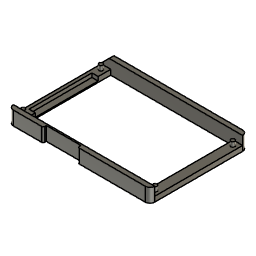
ScreenBezel v5 (Autodesk Fusion 360 design; units mm, degrees)
Autodesk Fusion 360 part; units mm, degrees
sketch "Sketch1" plane through (0, 0, 0) normal (0, 0, 1) x (1, 0, 0)
  line L0 (-50, 25) -> (28, 25)
  line L1 (28, 25) -> (28, -31)
  line L2 (28, -31) -> (-50, -31)
  line L3 (-50, -31) -> (-50, 25)
  line L4 (-55, 30) -> (30, 30)
  line L5 (30, 30) -> (30, -35)
  line L6 (30, -35) -> (-55, -35)
  line L7 (-55, -35) -> (-55, 30)
  dimension "d1" = 78
  dimension "d2" = 56
  constraint horizontal L0
  constraint vertical L1
  constraint horizontal L2
  constraint vertical L3
  constraint horizontal L4
  constraint vertical L5
  constraint horizontal L6
  constraint vertical L7
  measures "d1" distance of L0.start L0.end
  measures "d2" distance of L0.start L2.end
extrude "Extrude1" add sketch "Sketch1" along normal blind 3
sketch "Sketch2" plane through (0, 0, 3) normal (0, 0, 1) x (-1, 0, 0)
  line L0 (-28, 31) -> (50, 31)
  line L1 (50, 31) -> (50, -25)
  line L2 (50, -25) -> (-28, -25)
  line L3 (-28, -25) -> (-28, 31)
  line L4 (55, 35) -> (-30, 35)
  line L5 (-30, 35) -> (-30, -30)
  line L6 (-30, -30) -> (55, -30)
  line L7 (55, -30) -> (55, 35)
  line L8 (50, -25) -> (-28, -25)
  line L9 (-28, -25) -> (-28, -30)
  line L10 (-28, -30) -> (50, -30)
  line L11 (50, -30) -> (50, -25)
  line L12 (-28, 31) -> (50, 31)
  line L13 (50, 31) -> (50, 35)
  line L14 (50, 35) -> (-28, 35)
  line L15 (-28, 35) -> (-28, 31)
  constraint horizontal L8
  constraint vertical L9
  constraint horizontal L10
  constraint vertical L11
  constraint coincident L6 L9.end
  constraint coincident L1.end L2.start
  constraint horizontal L12
  constraint vertical L13
  constraint horizontal L14
  constraint vertical L15
  constraint coincident L4 L13.end
  constraint coincident L0.start L3.end
extrude "Extrude2" add sketch "Sketch2" along normal blind 5 contours L0 L4 L12 L13 L14 L15 | L2 L6 L8 L9 L10 L11
extrude "Extrude3" add 1 faces at (30, 8.3333, 1) along direction (1, 0, 0) blind 4
extrude "Extrude4" add 1 faces at (-55, -13.3333, 1) along direction (-1, 0, 0) blind 1
sketch "Sketch3" plane through (0, 0, 3) normal (0, 0, 1) x (-1, 0, 0)
  line L0 (50, 35) -> (50, 31)
  line L1 (50, 31) -> (50, -25)
  line L2 (50, -25) -> (50, -30)
  line L3 (50, -30) -> (56, -30)
  line L4 (56, -30) -> (56, 35)
  line L5 (56, 35) -> (50, 35)
  circle A0 centre (53, -21.75) radius 1.25
  circle A1 centre (-31, -21.75) radius 1.25
  circle A2 centre (-31, 27.75) radius 1.25
  circle A3 centre (53, 27.75) radius 1.25
  dimension "d11" = 2.5
  dimension "d12" = 2.5
  dimension "d13" = 2.5
  dimension "d14" = 2.5
  measures "d11" diameter of A0
  measures "d12" diameter of A1
  measures "d13" diameter of A2
  measures "d14" diameter of A3
extrude "Extrude5" add sketch "Sketch3" along normal blind 3 contours A0 | A1 | A2 | A3
extrude "Extrude6" add 2 faces at (2, 28.3333, 8) (2, -32.3333, 8) along direction (0, 0, 1) blind 1
extrude "Extrude7" cut 1 faces at (-24, 30, 7) along direction (0, -1, 0) blind 2
extrude "Extrude8" cut 1 faces at (-24, -35, 5) along direction (0, 1, 0) blind 1
sketch "Sketch4" plane through (0, 0, 3) normal (0, 0, 1) x (-1, 0, 0)
  line L0 (56, 34) -> (50, 34)
  line L1 (50, 34) -> (50, 31)
  line L2 (50, 31) -> (50, -25)
  line L3 (50, -25) -> (50, -28)
  line L4 (50, -28) -> (56, -28)
  line L5 (56, -28) -> (56, 34)
  circle A0 centre (53, -21.75) radius 1.25
  circle A1 centre (53, 27.75) radius 1.25
  line L6 (50, -17) -> (54, -17)
  line L7 (54, -17) -> (54, 23)
  line L8 (54, 23) -> (50, 23)
  line L9 (50, 23) -> (50, -17)
  constraint horizontal L6
  constraint vertical L7
  constraint horizontal L8
  constraint vertical L9
  constraint coincident L2 L6.start
extrude "Extrude9" cut sketch "Sketch4" against normal blind 2.5 contours L2 L6 L7 L8 L9
extrude "Extrude10" add 2 faces at (-50, -32, 5) (-50, 26, 5) along direction (-1, 0, 0) up to surface end surface through (-56, -35, 0) normal (-1, 0, 0) offset 0
extrude "Extrude11" add 2 faces at (28, -32, 7) (28, 26, 5) along direction (1, 0, 0) up to surface end surface through (34, 30, 0) normal (1, 0, 0) offset 0
extrude "Extrude12" cut 2 faces at (4, 26, 9) (4, -33, 9) along direction (0, 0, -1) blind 0.5
chamfer "Chamfer1" distance 5 angle 45 1 edges at (-56, 26.5, 8.5)
fillet "Fillet4" radius 3 3 edges at (-56, -34, 4.25) (34, -34, 4.25) (34, 28, 4.25)
sketch "Sketch5" plane through (0, -34, 0) normal (0, -1, 0) x (1, 0, 0)
  line L0 (31, 0) -> (31, 8.5)
  line L1 (31, 8.5) -> (-53, 8.5)
  line L2 (-53, 8.5) -> (-53, 0)
  line L3 (-53, 0) -> (31, 0)
  line L4 (-56, 0) -> (-34, 0)
  line L5 (-34, 0) -> (-34, 10.214)
  line L6 (-34, 10.214) -> (-12, 10.214)
  line L7 (-12, 10.214) -> (-12, -0.4704)
  line L8 (-12, -0.4704) -> (-34, -0.4704)
  line L9 (-34, -0.4704) -> (-34, 0)
  point P0 (-56, 0)
  dimension "d40" = 90
  dimension "d41" = 22
  constraint coincident P0 L4.start
  constraint coincident L3 L4.end
  constraint perpendicular L5 L6
  constraint perpendicular L3 L7
  constraint perpendicular L5 L8
  constraint perpendicular L3 L9
  measures "d40" angle of L4 L5
  measures "d41" distance of L5.end L6.end
extrude "Extrude13" cut sketch "Sketch5" against normal blind 2 contours L1 L3 L5 L7
fillet "Fillet5" radius 1 2 edges at (-34, -34, 4.25) (-12, -34, 4.25)
extrude "Extrude14" add 1 faces at (-54, 7.3331, 0) along direction (0, 0, -1) blind 0.25
